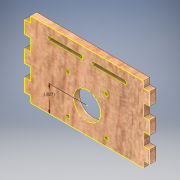
# Autodesk Inventor part: VerticalSupport
Saved by Autodesk Inventor 2019 (Build 230136000, 136)
## iProperties
Created: 2019-01-17
Part Number: VerticalSupport
Material: Wood (Birch)
Document SubType Name: Modeling
Designer: nxgam
Density: 0.55 g/cm^3
Appearance: Birch - Natural Polished
Mass: 14.8331 g
Surface Area: 136.304 cm^2
Volume: 26.9693 cm^3
Author: nxgam
Autodesk Inventor part; units mm, degrees
ref_plane "YZ Plane" through (0, 0, 0) normal (1, 0, 0) x (0, 1, 0)
ref_plane "XZ Plane" through (0, 0, 0) normal (0, 1, 0) x (-1, 0, 0)
ref_plane "XY Plane" through (0, 0, 0) normal (0, 0, 1) x (1, 0, 0)
sketch "Sketch1" plane through (0, 0, 0) normal (0, 0, 1) x (1, 0, 0)
  line L0 (45.72, 0) -> (45.72, 60.96)
  line L1 (45.72, 60.96) -> (-45.72, 60.96)
  line L2 (-45.72, 60.96) -> (-45.72, 9.301)
  line L3 (-45.72, 5.08) -> (-50.8, 5.08)
  line L4 (-50.8, 5.08) -> (-50.8, 15.24)
  line L5 (-50.8, 15.24) -> (-45.72, 15.24)
  line L6 (-45.72, 15.24) -> (-45.72, 5.08)
  line L7 (-45.72, 25.4) -> (-50.8, 25.4)
  line L8 (-50.8, 25.4) -> (-50.8, 35.56)
  line L9 (-50.8, 35.56) -> (-45.72, 35.56)
  line L10 (-45.72, 35.56) -> (-45.72, 25.4)
  line L11 (-45.72, 45.72) -> (-50.8, 45.72)
  line L12 (-50.8, 45.72) -> (-50.8, 55.88)
  line L13 (-50.8, 55.88) -> (-45.72, 55.88)
  line L14 (-45.72, 55.88) -> (-45.72, 45.72)
  line L15 (0, 60.96) -> (0, 0) construction
  line L16 (45.72, 60.96) -> (45.72, 0)
  line L17 (45.72, 5.08) -> (50.8, 5.08)
  line L18 (50.8, 5.08) -> (50.8, 15.24)
  line L19 (50.8, 15.24) -> (45.72, 15.24)
  line L20 (45.72, 15.24) -> (45.72, 5.08)
  line L21 (45.72, 25.4) -> (50.8, 25.4)
  line L22 (50.8, 25.4) -> (50.8, 35.56)
  line L23 (50.8, 35.56) -> (45.72, 35.56)
  line L24 (45.72, 35.56) -> (45.72, 25.4)
  line L25 (45.72, 45.72) -> (50.8, 45.72)
  line L26 (50.8, 45.72) -> (50.8, 55.88)
  line L27 (50.8, 55.88) -> (45.72, 55.88)
  line L28 (45.72, 55.88) -> (45.72, 45.72)
  line L29 (-45.72, 5.08) -> (-45.72, 0)
  line L30 (-45.72, 0) -> (45.72, 0)
  line L31 (45.72, 60.96) -> (-45.72, 60.96)
  line L32 (-45.72, 60.96) -> (-45.72, 0)
  line L33 (-45.72, 0) -> (45.72, 0)
  line L34 (45.72, 0) -> (45.72, 60.96)
  dimension "d0" = 91.44
  dimension "d2" = 10.16
  dimension "d3" = 5.08
  dimension "d7" = 20.32
  dimension "d14" = 5.08
  dimension "d15" = 60.96
  constraints: 70 end point, 12 symmetric about line, 5 parallel, 4 perpendicular, 3 vertical, 2 horizontal, 2 midpoint, 2 point on line, 1 coincident, 16 other
  measures "d0" distance of L1.end L0.end
  measures "d2" distance of L3.end L4.end
  measures "d3" distance of L4.end L5.end
  measures "d7" distance of L3.start L7.start
  measures "d14" distance of L3.start L29.end
  measures "d15" distance between parallel lines of L30 L1
extrude "Extrusion2" add sketch "Sketch1" along normal blind 5.08
sketch "Sketch2" plane through (0, 0, 0) normal (0, 0, -1) x (-1, 0, 0)
  circle A0 centre (-15.5, 5.5) radius 1.5 projected
  circle A1 centre (15.5, 36.5) radius 1.5 projected
  circle A2 centre (-15.5, 36.5) radius 1.5 projected
  circle A3 centre (15.5, 5.5) radius 1.5 projected
  line L0 (21, 3.175) -> (17.825, 0) projected
  line L1 (21, 38.825) -> (21, 3.175) projected
  line L2 (17.825, 42) -> (21, 38.825) projected
  line L3 (-17.825, 42) -> (17.825, 42) projected
  line L4 (-21, 38.825) -> (-17.825, 42) projected
  line L5 (-21, 3.175) -> (-21, 38.825) projected
  line L6 (-17.825, 0) -> (-21, 3.175) projected
  line L7 (17.825, 0) -> (-17.825, 0) projected
  circle A4 centre (0, 21) radius 11 projected
  circle A5 centre (0, 21) radius 2.25 projected
  point P0 (0, 0)
extrude "Extrusion3" cut sketch "Sketch2" against normal blind 25.4 contours A0 | A1 | A2 | A3 | A4 | A5
sketch "Sketch4" plane through (0, 0, 5.08) normal (0, 0, 1) x (1, 0, 0)
  line L0 (0, 0) -> (0, 60.96) construction
  line L1 (45.72, 60.96) -> (-45.72, 60.96) construction
  line L2 (-30.48, 52.75) -> (-5.08, 52.75) construction
  line L3 (-30.48, 51.25) -> (-5.08, 51.25)
  line L4 (-5.08, 54.25) -> (-30.48, 54.25)
  arc A0 (-30.48, 54.25) -> (-30.48, 51.25) centre (-30.48, 52.75) ccw
  arc A1 (-5.08, 51.25) -> (-5.08, 54.25) centre (-5.08, 52.75) ccw
  line L5 (30.48, 52.75) -> (5.08, 52.75) construction
  line L6 (30.48, 51.25) -> (5.08, 51.25)
  line L7 (5.08, 54.25) -> (30.48, 54.25)
  arc A2 (30.48, 51.25) -> (30.48, 54.25) centre (30.48, 52.75) ccw
  arc A3 (5.08, 54.25) -> (5.08, 51.25) centre (5.08, 52.75) ccw
  circle A4 centre (0, 21) radius 11 projected
  line L8 (-11, 21) -> (0, 21)
  point P0 (-17.78, 52.75)
  point P1 (17.78, 52.75)
  dimension "d25" = 3
  dimension "d26" = 25.4
  dimension "d28" = 17.78
  dimension "d31" = 31.75
  constraints: 20 end point, 8 point on circle, 7 symmetric about line, 4 centre point, 4 tangent, 2 horizontal, 2 midpoint, 1 horizontal alignment, 1 parallel, 3 other
  measures "d25" diameter of A1
  measures "d26" distance of L2.start L2.end
  measures "d28" distance from line of L0 point (-17.78, 52.75)
  measures "d31" distance between parallel lines of L2 L8
extrude "Extrusion5" cut sketch "Sketch4" against normal blind 25.4 contours A0 L4 A1 L3 | L6 A3 L7 A2
sketch "Sketch5" plane through (0, 0, 5.08) normal (0, 0, 1) x (1, 0, 0)
  arc A0 (-5.08, 51.25) -> (-5.08, 54.25) centre (-5.08, 52.75) ccw projected
  line L0 (-5.08, 51.25) -> (-30.48, 51.25) projected
  arc A1 (-30.48, 54.25) -> (-30.48, 51.25) centre (-30.48, 52.75) ccw projected
  line L1 (-30.48, 54.25) -> (-5.08, 54.25) projected
  arc A2 (30.48, 51.25) -> (30.48, 54.25) centre (30.48, 52.75) ccw projected
  line L2 (30.48, 51.25) -> (5.08, 51.25) projected
  arc A3 (5.08, 54.25) -> (5.08, 51.25) centre (5.08, 52.75) ccw projected
  line L3 (5.08, 54.25) -> (30.48, 54.25) projected
  circle A4 centre (-15.5, 5.5) radius 1.5 projected
  circle A5 centre (-15.5, 36.5) radius 1.5 projected
  circle A6 centre (15.5, 5.5) radius 1.5 projected
  circle A7 centre (15.5, 36.5) radius 1.5 projected
  circle A8 centre (0, 21) radius 11 projected
  line L4 (50.8, 25.4) -> (50.8, 35.56) projected
  line L5 (50.8, 35.56) -> (45.72, 35.56) projected
  line L6 (45.72, 35.56) -> (45.72, 45.72) projected
  line L7 (45.72, 45.72) -> (50.8, 45.72) projected
  line L8 (50.8, 45.72) -> (50.8, 55.88) projected
  line L9 (50.8, 55.88) -> (45.72, 55.88) projected
  line L10 (45.72, 55.88) -> (45.72, 60.96) projected
  line L11 (45.72, 60.96) -> (-45.72, 60.96) projected
  line L12 (-45.72, 60.96) -> (-45.72, 55.88) projected
  line L13 (-45.72, 55.88) -> (-50.8, 55.88) projected
  line L14 (-50.8, 55.88) -> (-50.8, 45.72) projected
  line L15 (-50.8, 45.72) -> (-45.72, 45.72) projected
  line L16 (-45.72, 45.72) -> (-45.72, 35.56) projected
  line L17 (-45.72, 35.56) -> (-50.8, 35.56) projected
  line L18 (-50.8, 35.56) -> (-50.8, 25.4) projected
  line L19 (-50.8, 25.4) -> (-45.72, 25.4) projected
  line L20 (-45.72, 25.4) -> (-45.72, 15.24) projected
  line L21 (-45.72, 15.24) -> (-50.8, 15.24) projected
  line L22 (-50.8, 15.24) -> (-50.8, 5.08) projected
  line L23 (-50.8, 5.08) -> (-45.72, 5.08) projected
  line L24 (-45.72, 5.08) -> (-45.72, 0) projected
  line L25 (-45.72, 0) -> (45.72, 0) projected
  line L26 (45.72, 0) -> (45.72, 5.08) projected
  line L27 (45.72, 5.08) -> (50.8, 5.08) projected
  line L28 (50.8, 5.08) -> (50.8, 15.24) projected
  line L29 (50.8, 15.24) -> (45.72, 15.24) projected
  line L30 (45.72, 15.24) -> (45.72, 25.4) projected
  line L31 (45.72, 25.4) -> (50.8, 25.4) projected
  point P0 (0, 0)
  dimension "d32" = 21
  measures "d32" distance from line of L25 A8.centre
equation "\"d7\" = 2 * d2"
body "Solid2"
